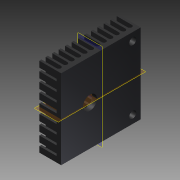
# Autodesk Inventor part: D-040
Saved by Autodesk Inventor 2015 (Build 190159000, 159)
## iProperties
Company: MARCHA TECHNOLOGY
Created: 2013-09-29
Part Number: D-040
Document SubType Name: Modeling
Designer: O.Martin
Density: 1 g/cm^3
Mass: 6.96628 g
Surface Area: 115.125 cm^2
Volume: 6.96628 cm^3
Project: WITBOXprinter_K01
Description: DISIPADOR
Stock Number: 28655
Material: Generic
Appearance: Rubber - Black - Version 1.1
Author: O.Martin
Autodesk Inventor part; units mm, degrees
ref_plane "YZ Plane" through (0, 0, 0) normal (1, 0, 0) x (0, 1, 0)
sketch "Boceto1" plane through (0, 0, 0) normal (0, 0, 1) x (1, 0, 0)
  line L0 (-11, -20) -> (0, -20)
  line L1 (0, -20) -> (0, 20)
  line L2 (0, 20) -> (-11, 20)
  line L3 (-11, 20) -> (-11, -20)
  line L4 (-11, -18.9) -> (-3.3705, -18.9)
  line L5 (-3.3705, -18.9) -> (-3.3705, -16.759)
  line L6 (-3.3705, -16.759) -> (-11, -16.759)
  line L7 (-11, -16.759) -> (-11, -18.9)
  circle A0 centre (-3.3705, -17.8295) radius 1.0705
  point P0 (0, 0)
  point P1 (0, 0)
  dimension "d4" = 2.141
  dimension "d0" = 40
  dimension "d1" = 11
  dimension "d2" = 1.1
  dimension "d3" = 2.3
  constraints: 16 end point, 4 parallel, 2 horizontal, 2 midpoint, 2 perpendicular, 1 coincident, 1 point on line, 1 vertical alignment, 2 other
  measures "d0" distance of L0.end L1.end
  measures "d1" distance of L1.end L2.end
  measures "d2" distance between parallel lines of L0 L4
extrude "Extrusión1" add sketch "Boceto1" along normal mid plane 40
extrude "Extrusión2" cut sketch "Boceto1" along normal through all both and the other way through all contours L3 L6 A0 L4 | A0 L5 | L5 A0
pattern_linear "Patrón rectangular1" count 12 spacing 3.241 along (0, 1, 0) of "Extrusión2"
sketch "Boceto2" plane through (-11, 20, 20) normal (0, 1, 0) x (1, 0, 0)
  line L0 (0, 0) -> (11, 0) projected
  line L1 (0, 40) -> (0, 0) projected
  line L2 (0, 3) -> (8.7, 3)
  line L3 (8.7, 3) -> (8.7, 4.625)
  line L4 (8.7, 4.625) -> (0, 4.625)
  line L5 (0, 4.625) -> (0, 3)
  line L6 (8.7, 0) -> (7.6295, 0) projected
  dimension "d12" = 3
  dimension "d13" = 1.625
  constraints: 8 end point, 2 parallel, 1 horizontal, 1 perpendicular, 1 point on line, 1 vertical alignment
  measures "d12" distance between parallel lines of L0 L2
  measures "d13" distance of L2.end L3.end
extrude "Extrusión3" cut sketch "Boceto2" against normal through all
pattern_linear "Patrón rectangular3" count 8 spacing 4.65 along (0, 0, -1) of "Extrusión3"
sketch "Boceto3" plane through (0, -20, 20) normal (1, 0, 0) x (0, 0, -1)
  line L0 (40, 40) -> (0, 40) projected
  line L1 (36, 36) -> (4, 36) construction
  line L2 (9.275, 30.269) -> (12.3, 30.269) construction
  point P0 (20, 36)
  point P1 (20, 40)
  dimension "d22" = 32
  dimension "d23" = 4
  constraints: 2 coincident, 2 end point, 2 midpoint, 1 parallel, 1 vertical alignment
  measures "d22" distance of L1.start L1.end
  measures "d23" distance between parallel lines of L0 L1
hole "Agujero1" at (0, 16, -16) at (0, 16, 16) direction (-1, 0, 0) diameter 3.5 end through all
sketch "Boceto5" plane through (0, -20, 20) normal (1, 0, 0) x (0, 0, -1)
  line L0 (40, 40) -> (0, 40) projected
  circle A0 centre (20, 14.5) radius 3.5
  point P0 (20, 40)
  dimension "d36" = 7
  dimension "d37" = 25.5
  constraints: 1 centre point, 1 midpoint, 1 vertical alignment
  measures "d36" diameter of A0
  measures "d37" distance from line of L0 A0.centre
extrude "Extrusión5" cut sketch "Boceto5" against normal through all
body "Solid1"
